Autodesk Fusion 360 part; units mm, degrees
note: some values were not read from the file. Set by a fixed rule: which sketch regions a step uses.
(part 2 of 2)
sketch "Sketch12" plane through (0, 70, 0) normal (0, 1, 0) x (-1, 0, 0)
  line L0 (-22.9298, -48.3019) -> (-17.9408, -50.3684)
  line L1 (-17.9408, -50.3684) -> (-19.1654, -53.3248)
  line L2 (-19.1654, -53.3248) -> (-19.6358, -53.13)
  arc A0 (-23.684, -51.4532) -> (-19.6358, -53.13) centre (-21.5833, -52.1068) ccw
  line L3 (-23.684, -51.4532) -> (-24.1544, -51.2583)
  line L4 (-24.1544, -51.2583) -> (-22.9298, -48.3019)
  line L5 (22.9298, 48.3019) -> (17.9408, 50.3684)
  line L6 (17.9408, 50.3684) -> (19.1654, 53.3248)
  line L7 (19.1654, 53.3248) -> (19.6358, 53.13)
  arc A1 (23.684, 51.4532) -> (19.6358, 53.13) centre (21.5833, 52.1068) ccw
  line L8 (23.684, 51.4532) -> (24.1544, 51.2583)
  line L9 (24.1544, 51.2583) -> (22.9298, 48.3019)
  line L10 (-17.9408, 50.3684) -> (-22.9298, 48.3019)
  line L11 (-22.9298, 48.3019) -> (-24.1544, 51.2583)
  line L12 (-24.1544, 51.2583) -> (-23.684, 51.4532)
  arc A2 (-19.6358, 53.13) -> (-23.684, 51.4532) centre (-21.5833, 52.1068) ccw
  line L13 (-19.6358, 53.13) -> (-19.1654, 53.3248)
  line L14 (-19.1654, 53.3248) -> (-17.9408, 50.3684)
  line L15 (-48.3019, 22.9298) -> (-50.3684, 17.9408)
  line L16 (-50.3684, 17.9408) -> (-53.3248, 19.1654)
  line L17 (-53.3248, 19.1654) -> (-53.13, 19.6358)
  arc A3 (-51.4532, 23.684) -> (-53.13, 19.6358) centre (-52.1068, 21.5833) ccw
  line L18 (-51.4532, 23.684) -> (-51.2583, 24.1544)
  line L19 (-51.2583, 24.1544) -> (-48.3019, 22.9298)
  line L20 (48.3019, -22.9298) -> (50.3684, -17.9408)
  line L21 (50.3684, -17.9408) -> (53.3248, -19.1654)
  line L22 (53.3248, -19.1654) -> (53.13, -19.6358)
  arc A4 (51.4532, -23.684) -> (53.13, -19.6358) centre (52.1068, -21.5833) ccw
  line L23 (51.4532, -23.684) -> (51.2583, -24.1544)
  line L24 (51.2583, -24.1544) -> (48.3019, -22.9298)
  line L25 (50.3684, 17.9408) -> (48.3019, 22.9298)
  line L26 (48.3019, 22.9298) -> (51.2583, 24.1544)
  line L27 (51.2583, 24.1544) -> (51.4532, 23.684)
  arc A5 (53.13, 19.6358) -> (51.4532, 23.684) centre (52.1068, 21.5833) ccw
  line L28 (53.13, 19.6358) -> (53.3248, 19.1654)
  line L29 (53.3248, 19.1654) -> (50.3684, 17.9408)
  line L30 (-2.1909, -56.6) -> (-2.7, -56.6)
  line L31 (-2.7, -56.6) -> (-2.7, -53.4)
  line L32 (-2.7, -53.4) -> (2.7, -53.4)
  line L33 (2.7, -53.4) -> (2.7, -56.6)
  line L34 (2.7, -56.6) -> (2.1909, -56.6)
  arc A6 (-2.1909, -56.6) -> (2.1909, -56.6) centre (0, -56.4) ccw
  line L35 (39.6687, 35.8503) -> (35.8503, 39.6687)
  line L36 (35.8503, 39.6687) -> (38.1131, 41.9314)
  line L37 (38.1131, 41.9314) -> (38.4731, 41.5714)
  arc A7 (41.5714, 38.4731) -> (38.4731, 41.5714) centre (39.8808, 39.8808) ccw
  line L38 (41.5714, 38.4731) -> (41.9314, 38.1131)
  line L39 (41.9314, 38.1131) -> (39.6687, 35.8503)
  line L40 (17.9408, -50.3684) -> (22.9298, -48.3019)
  line L41 (22.9298, -48.3019) -> (24.1544, -51.2583)
  line L42 (24.1544, -51.2583) -> (23.684, -51.4532)
  arc A8 (19.6358, -53.13) -> (23.684, -51.4532) centre (21.5833, -52.1068) ccw
  line L43 (19.6358, -53.13) -> (19.1654, -53.3248)
  line L44 (19.1654, -53.3248) -> (17.9408, -50.3684)
  line L45 (2.7, 53.4) -> (-2.7, 53.4)
  line L46 (-2.7, 53.4) -> (-2.7, 56.6)
  line L47 (-2.7, 56.6) -> (-2.1909, 56.6)
  arc A9 (2.1909, 56.6) -> (-2.1909, 56.6) centre (0, 56.4) ccw
  line L48 (2.1909, 56.6) -> (2.7, 56.6)
  line L49 (2.7, 56.6) -> (2.7, 53.4)
  line L50 (-35.8503, 39.6687) -> (-39.6687, 35.8503)
  line L51 (-39.6687, 35.8503) -> (-41.9314, 38.1131)
  line L52 (-41.9314, 38.1131) -> (-41.5714, 38.4731)
  arc A10 (-38.4731, 41.5714) -> (-41.5714, 38.4731) centre (-39.8808, 39.8808) ccw
  line L53 (-38.4731, 41.5714) -> (-38.1131, 41.9314)
  line L54 (-38.1131, 41.9314) -> (-35.8503, 39.6687)
  line L55 (-50.3684, -17.9408) -> (-48.3019, -22.9298)
  line L56 (-48.3019, -22.9298) -> (-51.2583, -24.1544)
  line L57 (-51.2583, -24.1544) -> (-51.4532, -23.684)
  arc A11 (-53.13, -19.6358) -> (-51.4532, -23.684) centre (-52.1068, -21.5833) ccw
  line L58 (-53.13, -19.6358) -> (-53.3248, -19.1654)
  line L59 (-53.3248, -19.1654) -> (-50.3684, -17.9408)
  line L60 (35.8503, -39.6687) -> (39.6687, -35.8503)
  line L61 (39.6687, -35.8503) -> (41.9314, -38.1131)
  line L62 (41.9314, -38.1131) -> (41.5714, -38.4731)
  arc A12 (38.4731, -41.5714) -> (41.5714, -38.4731) centre (39.8808, -39.8808) ccw
  line L63 (38.4731, -41.5714) -> (38.1131, -41.9314)
  line L64 (38.1131, -41.9314) -> (35.8503, -39.6687)
  line L65 (53.4, -2.7) -> (53.4, 2.7)
  line L66 (53.4, 2.7) -> (56.6, 2.7)
  line L67 (56.6, 2.7) -> (56.6, 2.1909)
  arc A13 (56.6, -2.1909) -> (56.6, 2.1909) centre (56.4, 0) ccw
  line L68 (56.6, -2.1909) -> (56.6, -2.7)
  line L69 (56.6, -2.7) -> (53.4, -2.7)
  circle A14 centre (0, 0) radius 51
  line L70 (-53.4, 2.7) -> (-53.4, -2.7)
  line L71 (-53.4, -2.7) -> (-56.6, -2.7)
  line L72 (-56.6, -2.7) -> (-56.6, -2.1909)
  arc A15 (-56.6, 2.1909) -> (-56.6, -2.1909) centre (-56.4, 0) ccw
  line L73 (-56.6, 2.1909) -> (-56.6, 2.7)
  line L74 (-56.6, 2.7) -> (-53.4, 2.7)
  line L75 (-39.6687, -35.8503) -> (-35.8503, -39.6687)
  line L76 (-35.8503, -39.6687) -> (-38.1131, -41.9314)
  line L77 (-38.1131, -41.9314) -> (-38.4731, -41.5714)
  arc A16 (-41.5714, -38.4731) -> (-38.4731, -41.5714) centre (-39.8808, -39.8808) ccw
  line L78 (-41.5714, -38.4731) -> (-41.9314, -38.1131)
  line L79 (-41.9314, -38.1131) -> (-39.6687, -35.8503)
  line L80 (0, 0) -> (0, -9) construction
  line L81 (0, 0) -> (-7, 0) construction
  line L82 (0, 0) -> (36.0624, -36.0624) construction
  line L83 (0, 0) -> (51, 0) construction
  line L84 (36.0624, -36.0624) -> (33.234, -33.234)
  circle A17 centre (33.234, -33.234) radius 1.5
  line L85 (38.1213, -33.8787) -> (33.1716, -28.9289)
  line L86 (33.8787, -38.1213) -> (28.9289, -33.1716)
  line L87 (33.1716, -28.9289) -> (28.9289, -33.1716)
  circle A18 centre (-33.234, -33.234) radius 1.5
  line L88 (-33.1716, -28.9289) -> (-28.9289, -33.1716)
  line L89 (-36.0624, -36.0624) -> (-33.234, -33.234)
  line L90 (-33.8787, -38.1213) -> (-28.9289, -33.1716)
  line L91 (-38.1213, -33.8787) -> (-33.1716, -28.9289)
  line L92 (0, 0) -> (-36.0624, -36.0624) construction
  circle A19 centre (33.234, 33.234) radius 1.5
  line L93 (33.1716, 28.9289) -> (28.9289, 33.1716)
  line L94 (33.8787, 38.1213) -> (28.9289, 33.1716)
  line L95 (38.1213, 33.8787) -> (33.1716, 28.9289)
  line L96 (-33.1716, 28.9289) -> (-28.9289, 33.1716)
  line L97 (-33.8787, 38.1213) -> (-28.9289, 33.1716)
  circle A20 centre (-33.234, 33.234) radius 1.5
  line L98 (-38.1213, 33.8787) -> (-33.1716, 28.9289)
  circle A21 centre (0, 0) radius 60
  dimension "d133" = 45
  dimension "d134" = 4
  dimension "d135" = 3
  dimension "d138" = 7
  dimension "d139" = 7
  constraint coincident A14.centre L80.start
  constraint vertical L80
  constraint perpendicular L80 L81
  constraint horizontal L83
  constraint parallel L82 L84
  constraint coincident L84.end A17.centre
  constraint coincident A14 L85.start
  constraint coincident A14 L86.start
  constraint perpendicular L86 L87
  constraint symmetric L80 A14.centre L81.start
  constraint symmetric L80 L82.end L89.start
  constraint symmetric L80 L84.end A18.centre
  constraint symmetric L80 A17 A18
  constraint symmetric L80 L85.start L91.start
  constraint symmetric L80 L86.start L90.start
  constraint symmetric L80 L85.end L88.start
  constraint symmetric L80 L86.end L88.end
  constraint symmetric L81 A17 A19
  constraint symmetric L81 L85.start L95.start
  constraint symmetric L81 L86.start L94.start
  constraint symmetric L81 L85.end L93.start
  constraint symmetric L81 L86.end L93.end
  constraint symmetric L81 L88.start L96.start
  constraint symmetric L81 L88.end L96.end
  constraint symmetric L81 L91.start L98.start
  constraint symmetric L81 A18 A20
  constraint symmetric L81 L90.start L97.start
  measures "d133" angle of L82 L83
  measures "d134" distance of L82.end L84.end
  measures "d135" diameter of A17
  measures "d138" distance of L85.start L85.end
  measures "d139" distance of L86.start L86.end
extrude "Extrude15" add sketch "Sketch12" against normal blind 9 contours A14 L93 L94 L95 | A14 L85 L86 L87 | A14 L96 L97 L98 | A14 L88 L90 L91 bodies 1
sketch "Sketch13" plane through (0, 70, 0) normal (0, 1, 0) x (-1, 0, 0)
  line L0 (-28.9289, 33.1716) -> (-33.8787, 38.1213)
  arc A0 (33.8787, 38.1213) -> (-33.8787, 38.1213) centre (0, 0) ccw
  line L1 (33.8787, 38.1213) -> (28.9289, 33.1716)
  line L2 (33.1716, 28.9289) -> (38.1213, 33.8787)
  arc A1 (38.1213, -33.8787) -> (38.1213, 33.8787) centre (0, 0) ccw
  line L3 (38.1213, -33.8787) -> (33.1716, -28.9289)
  line L4 (28.9289, -33.1716) -> (33.8787, -38.1213)
  arc A2 (-33.8787, -38.1213) -> (33.8787, -38.1213) centre (0, 0) ccw
  line L5 (-33.8787, -38.1213) -> (-28.9289, -33.1716)
  line L6 (-33.1716, -28.9289) -> (-38.1213, -33.8787)
  arc A3 (-38.1213, 33.8787) -> (-38.1213, -33.8787) centre (0, 0) ccw
  line L7 (-38.1213, 33.8787) -> (-33.1716, 28.9289)
  circle A4 centre (-33.234, 33.234) radius 1.5
  circle A5 centre (-33.234, -33.234) radius 1.5
  circle A6 centre (33.234, 33.234) radius 1.5
  circle A7 centre (33.234, -33.234) radius 1.5
  line L8 (-22.9298, -48.3019) -> (-17.9408, -50.3684)
  line L9 (-17.9408, -50.3684) -> (-19.1654, -53.3248)
  line L10 (-19.1654, -53.3248) -> (-19.6358, -53.13)
  arc A8 (-23.684, -51.4532) -> (-19.6358, -53.13) centre (-21.5833, -52.1068) ccw
  line L11 (-23.684, -51.4532) -> (-24.1544, -51.2583)
  line L12 (-24.1544, -51.2583) -> (-22.9298, -48.3019)
  line L13 (22.9298, 48.3019) -> (17.9408, 50.3684)
  line L14 (17.9408, 50.3684) -> (19.1654, 53.3248)
  line L15 (19.1654, 53.3248) -> (19.6358, 53.13)
  arc A9 (23.684, 51.4532) -> (19.6358, 53.13) centre (21.5833, 52.1068) ccw
  line L16 (23.684, 51.4532) -> (24.1544, 51.2583)
  line L17 (24.1544, 51.2583) -> (22.9298, 48.3019)
  line L18 (-17.9408, 50.3684) -> (-22.9298, 48.3019)
  line L19 (-22.9298, 48.3019) -> (-24.1544, 51.2583)
  line L20 (-24.1544, 51.2583) -> (-23.684, 51.4532)
  arc A10 (-19.6358, 53.13) -> (-23.684, 51.4532) centre (-21.5833, 52.1068) ccw
  line L21 (-19.6358, 53.13) -> (-19.1654, 53.3248)
  line L22 (-19.1654, 53.3248) -> (-17.9408, 50.3684)
  line L23 (-48.3019, 22.9298) -> (-50.3684, 17.9408)
  line L24 (-50.3684, 17.9408) -> (-53.3248, 19.1654)
  line L25 (-53.3248, 19.1654) -> (-53.13, 19.6358)
  arc A11 (-51.4532, 23.684) -> (-53.13, 19.6358) centre (-52.1068, 21.5833) ccw
  line L26 (-51.4532, 23.684) -> (-51.2583, 24.1544)
  line L27 (-51.2583, 24.1544) -> (-48.3019, 22.9298)
  line L28 (48.3019, -22.9298) -> (50.3684, -17.9408)
  line L29 (50.3684, -17.9408) -> (53.3248, -19.1654)
  line L30 (53.3248, -19.1654) -> (53.13, -19.6358)
  arc A12 (51.4532, -23.684) -> (53.13, -19.6358) centre (52.1068, -21.5833) ccw
  line L31 (51.4532, -23.684) -> (51.2583, -24.1544)
  line L32 (51.2583, -24.1544) -> (48.3019, -22.9298)
  line L33 (50.3684, 17.9408) -> (48.3019, 22.9298)
  line L34 (48.3019, 22.9298) -> (51.2583, 24.1544)
  line L35 (51.2583, 24.1544) -> (51.4532, 23.684)
  arc A13 (53.13, 19.6358) -> (51.4532, 23.684) centre (52.1068, 21.5833) ccw
  line L36 (53.13, 19.6358) -> (53.3248, 19.1654)
  line L37 (53.3248, 19.1654) -> (50.3684, 17.9408)
  line L38 (-2.1909, -56.6) -> (-2.7, -56.6)
  line L39 (-2.7, -56.6) -> (-2.7, -53.4)
  line L40 (-2.7, -53.4) -> (2.7, -53.4)
  line L41 (2.7, -53.4) -> (2.7, -56.6)
  line L42 (2.7, -56.6) -> (2.1909, -56.6)
  arc A14 (-2.1909, -56.6) -> (2.1909, -56.6) centre (0, -56.4) ccw
  line L43 (39.6687, 35.8503) -> (35.8503, 39.6687)
  line L44 (35.8503, 39.6687) -> (38.1131, 41.9314)
  line L45 (38.1131, 41.9314) -> (38.4731, 41.5714)
  arc A15 (41.5714, 38.4731) -> (38.4731, 41.5714) centre (39.8808, 39.8808) ccw
  line L46 (41.5714, 38.4731) -> (41.9314, 38.1131)
  line L47 (41.9314, 38.1131) -> (39.6687, 35.8503)
  line L48 (17.9408, -50.3684) -> (22.9298, -48.3019)
  line L49 (22.9298, -48.3019) -> (24.1544, -51.2583)
  line L50 (24.1544, -51.2583) -> (23.684, -51.4532)
  arc A16 (19.6358, -53.13) -> (23.684, -51.4532) centre (21.5833, -52.1068) ccw
  line L51 (19.6358, -53.13) -> (19.1654, -53.3248)
  line L52 (19.1654, -53.3248) -> (17.9408, -50.3684)
  line L53 (2.7, 53.4) -> (-2.7, 53.4)
  line L54 (-2.7, 53.4) -> (-2.7, 56.6)
  line L55 (-2.7, 56.6) -> (-2.1909, 56.6)
  arc A17 (2.1909, 56.6) -> (-2.1909, 56.6) centre (0, 56.4) ccw
  line L56 (2.1909, 56.6) -> (2.7, 56.6)
  line L57 (2.7, 56.6) -> (2.7, 53.4)
  line L58 (-35.8503, 39.6687) -> (-39.6687, 35.8503)
  line L59 (-39.6687, 35.8503) -> (-41.9314, 38.1131)
  line L60 (-41.9314, 38.1131) -> (-41.5714, 38.4731)
  arc A18 (-38.4731, 41.5714) -> (-41.5714, 38.4731) centre (-39.8808, 39.8808) ccw
  line L61 (-38.4731, 41.5714) -> (-38.1131, 41.9314)
  line L62 (-38.1131, 41.9314) -> (-35.8503, 39.6687)
  line L63 (-50.3684, -17.9408) -> (-48.3019, -22.9298)
  line L64 (-48.3019, -22.9298) -> (-51.2583, -24.1544)
  line L65 (-51.2583, -24.1544) -> (-51.4532, -23.684)
  arc A19 (-53.13, -19.6358) -> (-51.4532, -23.684) centre (-52.1068, -21.5833) ccw
  line L66 (-53.13, -19.6358) -> (-53.3248, -19.1654)
  line L67 (-53.3248, -19.1654) -> (-50.3684, -17.9408)
  line L68 (35.8503, -39.6687) -> (39.6687, -35.8503)
  line L69 (39.6687, -35.8503) -> (41.9314, -38.1131)
  line L70 (41.9314, -38.1131) -> (41.5714, -38.4731)
  arc A20 (38.4731, -41.5714) -> (41.5714, -38.4731) centre (39.8808, -39.8808) ccw
  line L71 (38.4731, -41.5714) -> (38.1131, -41.9314)
  line L72 (38.1131, -41.9314) -> (35.8503, -39.6687)
  line L73 (53.4, -2.7) -> (53.4, 2.7)
  line L74 (53.4, 2.7) -> (56.6, 2.7)
  line L75 (56.6, 2.7) -> (56.6, 2.1909)
  arc A21 (56.6, -2.1909) -> (56.6, 2.1909) centre (56.4, 0) ccw
  line L76 (56.6, -2.1909) -> (56.6, -2.7)
  line L77 (56.6, -2.7) -> (53.4, -2.7)
  line L78 (-53.4, 2.7) -> (-53.4, -2.7)
  line L79 (-53.4, -2.7) -> (-56.6, -2.7)
  line L80 (-56.6, -2.7) -> (-56.6, -2.1909)
  arc A22 (-56.6, 2.1909) -> (-56.6, -2.1909) centre (-56.4, 0) ccw
  line L81 (-56.6, 2.1909) -> (-56.6, 2.7)
  line L82 (-56.6, 2.7) -> (-53.4, 2.7)
  line L83 (-39.6687, -35.8503) -> (-35.8503, -39.6687)
  line L84 (-35.8503, -39.6687) -> (-38.1131, -41.9314)
  line L85 (-38.1131, -41.9314) -> (-38.4731, -41.5714)
  arc A23 (-41.5714, -38.4731) -> (-38.4731, -41.5714) centre (-39.8808, -39.8808) ccw
  line L86 (-41.5714, -38.4731) -> (-41.9314, -38.1131)
  line L87 (-41.9314, -38.1131) -> (-39.6687, -35.8503)
  circle A24 centre (0, 0) radius 60
  line L88 (-28.9289, -33.1716) -> (-33.1716, -28.9289)
  line L89 (-33.1716, 28.9289) -> (-28.9289, 33.1716)
  line L90 (28.9289, 33.1716) -> (33.1716, 28.9289)
  line L91 (33.1716, -28.9289) -> (28.9289, -33.1716)
  circle A25 centre (0, 0) radius 60
  constraint coincident A0.centre A1.centre
extrude "Extrude16" add sketch "Sketch13" along normal blind 3 separate body contours L0 A0 L1 L2 A1 L3 L4 A2 L5 L6 A3 L7 L88 L89 L90 L91 | L8 L9 L10 A8 L11 L12 | L13 L14 L15 A9 L16 L17 | L18 L19 L20 A10 L21 L22 | L23 L24 L25 A11 L26 L27 | L28 L29 L30 A12 L31 L32 | L33 L34 L35 A13 L36 L37 | L38 L39 L40 L41 L42 A14 | L43 L44 L45 A15 L46 L47 | L48 L49 L50 A16 L51 L52 | L53 L54 L55 A17 L56 L57 | L58 L59 L60 A18 L61 L62 | L63 L64 L65 A19 L66 L67 | L68 L69 L70 A20 L71 L72 | L73 L74 L75 A21 L76 L77 | L78 L79 L80 A22 L81 L82 | L83 L84 L85 A23 L86 L87 | A24 A25 makes body 2
sketch "Sketch14" plane through (0, 70, 0) normal (0, 1, 0) x (-1, 0, 0)
  circle A0 centre (-33.234, 33.234) radius 1.5
  circle A1 centre (-33.234, -33.234) radius 1.5
  circle A2 centre (33.234, 33.234) radius 1.5
  circle A3 centre (33.234, -33.234) radius 1.5
  line L0 (-22.9298, -48.3019) -> (-17.9408, -50.3684)
  line L1 (-17.9408, -50.3684) -> (-19.1654, -53.3248)
  line L2 (-19.1654, -53.3248) -> (-19.6358, -53.13)
  arc A4 (-23.684, -51.4532) -> (-19.6358, -53.13) centre (-21.5833, -52.1068) ccw
  line L3 (-23.684, -51.4532) -> (-24.1544, -51.2583)
  line L4 (-24.1544, -51.2583) -> (-22.9298, -48.3019)
  line L5 (22.9298, 48.3019) -> (17.9408, 50.3684)
  line L6 (17.9408, 50.3684) -> (19.1654, 53.3248)
  line L7 (19.1654, 53.3248) -> (19.6358, 53.13)
  arc A5 (23.684, 51.4532) -> (19.6358, 53.13) centre (21.5833, 52.1068) ccw
  line L8 (23.684, 51.4532) -> (24.1544, 51.2583)
  line L9 (24.1544, 51.2583) -> (22.9298, 48.3019)
  line L10 (-17.9408, 50.3684) -> (-22.9298, 48.3019)
  line L11 (-22.9298, 48.3019) -> (-24.1544, 51.2583)
  line L12 (-24.1544, 51.2583) -> (-23.684, 51.4532)
  arc A6 (-19.6358, 53.13) -> (-23.684, 51.4532) centre (-21.5833, 52.1068) ccw
  line L13 (-19.6358, 53.13) -> (-19.1654, 53.3248)
  line L14 (-19.1654, 53.3248) -> (-17.9408, 50.3684)
  line L15 (-48.3019, 22.9298) -> (-50.3684, 17.9408)
  line L16 (-50.3684, 17.9408) -> (-53.3248, 19.1654)
  line L17 (-53.3248, 19.1654) -> (-53.13, 19.6358)
  arc A7 (-51.4532, 23.684) -> (-53.13, 19.6358) centre (-52.1068, 21.5833) ccw
  line L18 (-51.4532, 23.684) -> (-51.2583, 24.1544)
  line L19 (-51.2583, 24.1544) -> (-48.3019, 22.9298)
  line L20 (48.3019, -22.9298) -> (50.3684, -17.9408)
  line L21 (50.3684, -17.9408) -> (53.3248, -19.1654)
  line L22 (53.3248, -19.1654) -> (53.13, -19.6358)
  arc A8 (51.4532, -23.684) -> (53.13, -19.6358) centre (52.1068, -21.5833) ccw
  line L23 (51.4532, -23.684) -> (51.2583, -24.1544)
  line L24 (51.2583, -24.1544) -> (48.3019, -22.9298)
  line L25 (50.3684, 17.9408) -> (48.3019, 22.9298)
  line L26 (48.3019, 22.9298) -> (51.2583, 24.1544)
  line L27 (51.2583, 24.1544) -> (51.4532, 23.684)
  arc A9 (53.13, 19.6358) -> (51.4532, 23.684) centre (52.1068, 21.5833) ccw
  line L28 (53.13, 19.6358) -> (53.3248, 19.1654)
  line L29 (53.3248, 19.1654) -> (50.3684, 17.9408)
  line L30 (-2.1909, -56.6) -> (-2.7, -56.6)
  line L31 (-2.7, -56.6) -> (-2.7, -53.4)
  line L32 (-2.7, -53.4) -> (2.7, -53.4)
  line L33 (2.7, -53.4) -> (2.7, -56.6)
  line L34 (2.7, -56.6) -> (2.1909, -56.6)
  arc A10 (-2.1909, -56.6) -> (2.1909, -56.6) centre (0, -56.4) ccw
  line L35 (39.6687, 35.8503) -> (35.8503, 39.6687)
  line L36 (35.8503, 39.6687) -> (38.1131, 41.9314)
  line L37 (38.1131, 41.9314) -> (38.4731, 41.5714)
  arc A11 (41.5714, 38.4731) -> (38.4731, 41.5714) centre (39.8808, 39.8808) ccw
  line L38 (41.5714, 38.4731) -> (41.9314, 38.1131)
  line L39 (41.9314, 38.1131) -> (39.6687, 35.8503)
  line L40 (17.9408, -50.3684) -> (22.9298, -48.3019)
  line L41 (22.9298, -48.3019) -> (24.1544, -51.2583)
  line L42 (24.1544, -51.2583) -> (23.684, -51.4532)
  arc A12 (19.6358, -53.13) -> (23.684, -51.4532) centre (21.5833, -52.1068) ccw
  line L43 (19.6358, -53.13) -> (19.1654, -53.3248)
  line L44 (19.1654, -53.3248) -> (17.9408, -50.3684)
  line L45 (2.7, 53.4) -> (-2.7, 53.4)
  line L46 (-2.7, 53.4) -> (-2.7, 56.6)
  line L47 (-2.7, 56.6) -> (-2.1909, 56.6)
  arc A13 (2.1909, 56.6) -> (-2.1909, 56.6) centre (0, 56.4) ccw
  line L48 (2.1909, 56.6) -> (2.7, 56.6)
  line L49 (2.7, 56.6) -> (2.7, 53.4)
  line L50 (-35.8503, 39.6687) -> (-39.6687, 35.8503)
  line L51 (-39.6687, 35.8503) -> (-41.9314, 38.1131)
  line L52 (-41.9314, 38.1131) -> (-41.5714, 38.4731)
  arc A14 (-38.4731, 41.5714) -> (-41.5714, 38.4731) centre (-39.8808, 39.8808) ccw
  line L53 (-38.4731, 41.5714) -> (-38.1131, 41.9314)
  line L54 (-38.1131, 41.9314) -> (-35.8503, 39.6687)
  line L55 (-50.3684, -17.9408) -> (-48.3019, -22.9298)
  line L56 (-48.3019, -22.9298) -> (-51.2583, -24.1544)
  line L57 (-51.2583, -24.1544) -> (-51.4532, -23.684)
  arc A15 (-53.13, -19.6358) -> (-51.4532, -23.684) centre (-52.1068, -21.5833) ccw
  line L58 (-53.13, -19.6358) -> (-53.3248, -19.1654)
  line L59 (-53.3248, -19.1654) -> (-50.3684, -17.9408)
  line L60 (35.8503, -39.6687) -> (39.6687, -35.8503)
  line L61 (39.6687, -35.8503) -> (41.9314, -38.1131)
  line L62 (41.9314, -38.1131) -> (41.5714, -38.4731)
  arc A16 (38.4731, -41.5714) -> (41.5714, -38.4731) centre (39.8808, -39.8808) ccw
  line L63 (38.4731, -41.5714) -> (38.1131, -41.9314)
  line L64 (38.1131, -41.9314) -> (35.8503, -39.6687)
  line L65 (53.4, -2.7) -> (53.4, 2.7)
  line L66 (53.4, 2.7) -> (56.6, 2.7)
  line L67 (56.6, 2.7) -> (56.6, 2.1909)
  arc A17 (56.6, -2.1909) -> (56.6, 2.1909) centre (56.4, 0) ccw
  line L68 (56.6, -2.1909) -> (56.6, -2.7)
  line L69 (56.6, -2.7) -> (53.4, -2.7)
  arc A18 (-33.8787, -38.1213) -> (33.8787, -38.1213) centre (0, 0) ccw
  line L70 (-33.8787, -38.1213) -> (-28.9289, -33.1716)
  line L71 (-28.9289, -33.1716) -> (-33.1716, -28.9289)
  line L72 (-33.1716, -28.9289) -> (-38.1213, -33.8787)
  arc A19 (-38.1213, 33.8787) -> (-38.1213, -33.8787) centre (0, 0) ccw
  line L73 (-38.1213, 33.8787) -> (-33.1716, 28.9289)
  line L74 (-33.1716, 28.9289) -> (-28.9289, 33.1716)
  line L75 (-28.9289, 33.1716) -> (-33.8787, 38.1213)
  arc A20 (33.8787, 38.1213) -> (-33.8787, 38.1213) centre (0, 0) ccw
  line L76 (33.8787, 38.1213) -> (28.9289, 33.1716)
  line L77 (28.9289, 33.1716) -> (33.1716, 28.9289)
  line L78 (33.1716, 28.9289) -> (38.1213, 33.8787)
  arc A21 (38.1213, -33.8787) -> (38.1213, 33.8787) centre (0, 0) ccw
  line L79 (38.1213, -33.8787) -> (33.1716, -28.9289)
  line L80 (33.1716, -28.9289) -> (28.9289, -33.1716)
  line L81 (28.9289, -33.1716) -> (33.8787, -38.1213)
  line L82 (-53.4, 2.7) -> (-53.4, -2.7)
  line L83 (-53.4, -2.7) -> (-56.6, -2.7)
  line L84 (-56.6, -2.7) -> (-56.6, -2.1909)
  arc A22 (-56.6, 2.1909) -> (-56.6, -2.1909) centre (-56.4, 0) ccw
  line L85 (-56.6, 2.1909) -> (-56.6, 2.7)
  line L86 (-56.6, 2.7) -> (-53.4, 2.7)
  line L87 (-39.6687, -35.8503) -> (-35.8503, -39.6687)
  line L88 (-35.8503, -39.6687) -> (-38.1131, -41.9314)
  line L89 (-38.1131, -41.9314) -> (-38.4731, -41.5714)
  arc A23 (-41.5714, -38.4731) -> (-38.4731, -41.5714) centre (-39.8808, -39.8808) ccw
  line L90 (-41.5714, -38.4731) -> (-41.9314, -38.1131)
  line L91 (-41.9314, -38.1131) -> (-39.6687, -35.8503)
  circle A24 centre (0, 0) radius 60
  line L92 (0, 0) -> (-49.8882, -33.3342) construction
  line L93 (0, 0) -> (60, 0) construction
  line L94 (0, 0) -> (-15, 0) construction
  line L95 (0, 0) -> (0, 10) construction
  line L96 (0, 0) -> (-49.8882, 33.3342) construction
  line L97 (0, 0) -> (49.8882, -33.3342) construction
  line L98 (0, 0) -> (49.8882, 33.3342) construction
  line L99 (42.405, 28.3341) -> (49.8882, 33.3342) construction
  line L100 (43.9243, 34.16) -> (53.9019, 40.8269)
  line L101 (53.9019, 40.8269) -> (58.3465, 34.1751)
  line L102 (58.3465, 34.1751) -> (48.3688, 27.5083)
  line L103 (58.3465, -34.1751) -> (48.3688, -27.5083)
  line L104 (53.9019, -40.8269) -> (58.3465, -34.1751)
  line L105 (43.9243, -34.16) -> (53.9019, -40.8269)
  line L106 (-43.9243, -34.16) -> (-53.9019, -40.8269)
  line L107 (-53.9019, -40.8269) -> (-58.3465, -34.1751)
  line L108 (-58.3465, -34.1751) -> (-48.3688, -27.5083)
  line L109 (-58.3465, 34.1751) -> (-48.3688, 27.5083)
  line L110 (-53.9019, 40.8269) -> (-58.3465, 34.1751)
  line L111 (-43.9243, 34.16) -> (-53.9019, 40.8269)
  line L112 (-49.8882, -33.3342) -> (-53.0062, -35.4176) construction
  circle A25 centre (-53.0062, -35.4176) radius 1.65
  circle A26 centre (-53.0062, 35.4176) radius 1.65
  circle A27 centre (53.0062, -35.4176) radius 1.65
  circle A28 centre (53.0062, 35.4176) radius 1.65
  dimension "d146" = 146.25
  dimension "d147" = 60
  dimension "d149" = 12
  dimension "d150" = 8
  dimension "d151" = 12
  dimension "d152" = 3.75
  dimension "d153" = 3.3
  constraint horizontal L93
  constraint coincident A18.centre A19.centre
  constraint parallel L93 L94
  constraint perpendicular L93 L95
  constraint symmetric A18.centre L94 A19.centre
  constraint symmetric L92.end L94 L96.end
  constraint symmetric A18.centre L95 A19.centre
  constraint symmetric L92.end L95 L97.end
  constraint symmetric L95 A18.centre A19.centre
  constraint symmetric L95 L96.end L98.end
  constraint coincident L98 L99.start
  constraint coincident A21 L99.start
  constraint perpendicular L100 L101
  constraint perpendicular L101 L102
  constraint symmetric L93 L100.start L105.start
  constraint symmetric L93 L100.end L104.start
  constraint symmetric L93 L101.end L103.start
  constraint symmetric L93 L102.end L103.end
  constraint symmetric L95 L100.start L111.start
  constraint symmetric L95 L100.end L110.start
  constraint symmetric L95 L101.end L109.start
  constraint symmetric L95 L102.end L109.end
  constraint symmetric L95 L103.start L107.end
  constraint symmetric L95 L103.end L108.end
  constraint symmetric L95 L104.start L106.end
  constraint symmetric L95 L105.start L106.start
  constraint perpendicular L107 L112
  constraint coincident L112.end A25.centre
  constraint symmetric L94 A25 A26
  constraint symmetric L95 A25 A27
  constraint symmetric L95 A26 A28
  measures "d146" angle of L92 L93
  measures "d147" distance of A18.centre L92.end
  measures "d149" distance of L100.start L100.end
  measures "d150" distance of L100.end L101.end
  measures "d151" distance of L101.end L102.end
  measures "d152" distance of L92.end L112.end
  measures "d153" diameter of A25
extrude "Extrude17" add sketch "Sketch14" against normal blind 9 contours A24 L100 L101 L102 | A24 L103 L104 L105 | A24 L109 L110 L111 | A24 L106 L107 L108 bodies 1
fillet "Fillet6" radius 3 16 edges at (28.9289, 65.5, 33.1716) (33.1716, 65.5, 28.9289) (28.9289, 65.5, -33.1716) (33.1716, 65.5, -28.9289) (33.8787, 65.5, -38.1213) (-38.1213, 65.5, -33.8787) (-33.1716, 65.5, -28.9289) (-28.9289, 65.5, -33.1716) (-33.8787, 65.5, -38.1213) (-28.9289, 65.5, 33.1716) (-33.8787, 65.5, 38.1213) (-33.1716, 65.5, 28.9289) (-38.1213, 65.5, 33.8787) (38.1213, 65.5, 33.8787) (33.8787, 65.5, 38.1213) (38.1213, 65.5, -33.8787) on bodies 1
fillet "Fillet7" radius 4 16 edges at (-53.9019, 65.5, 40.8269) (-58.3465, 65.5, 34.1751) (-47.5549, 65.5, 36.5859) (-51.9995, 65.5, 29.9342) (-58.3465, 65.5, -34.1751) (-51.9995, 65.5, -29.9342) (-53.9019, 65.5, -40.8269) (-47.5549, 65.5, -36.5859) (47.5549, 65.5, -36.5859) (53.9019, 65.5, -40.8269) (51.9995, 65.5, -29.9342) (58.3465, 65.5, -34.1751) (58.3465, 65.5, 34.1751) (51.9995, 65.5, 29.9342) (47.5549, 65.5, 36.5859) (53.9019, 65.5, 40.8269) on bodies 1
hidden bodies 2
equation "d8 = ( 31.75 / 2 ) * 1 mm"
equation "d14 = ( 76 / 2 ) * 1 mm"
equation "d36 = ( 360 / 32 ) * 1 deg"
equation "d51 = ( 360 / 32 ) * 1 deg"
equation "d152 = ( 7.5 / 2 ) * 1 mm"
